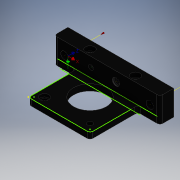
# Autodesk Inventor part: Part1
Saved by Autodesk Inventor 2016 SP1 (Build 200210100, 210)
## iProperties
Created: 2015-12-23
Part Number: Part1
Material: Generic
Document SubType Name: Modeling
Designer: Dirk Alferink
Density: 1 g/cm^3
Appearance: Smooth - Black
Author: Dirk Alferink
Autodesk Inventor part; units mm, degrees
ref_plane "YZ Plane" through (0, 0, 0) normal (1, 0, 0) x (0, 1, 0)
ref_plane "XZ Plane" through (0, 0, 0) normal (0, 1, 0) x (-1, 0, 0)
sketch "Sketch1" plane through (0, 0, 0) normal (0, 0, 1) x (1, 0, 0)
  line L0 (0, 0) -> (42, 0)
  line L1 (42, 0) -> (42, 42)
  line L2 (42, 42) -> (0, 42)
  line L3 (0, 42) -> (0, 0)
  dimension "d0" = 42
  dimension "d1" = 42
  constraints: 8 end point, 2 parallel, 1 horizontal, 1 perpendicular
  measures "d0" distance of L2.end L1.end
  measures "d1" distance of L1.end L0.end
extrude "Extrusion1" add sketch "Sketch1" along normal blind 4.3
sketch "Sketch2" plane through (0, 0, 4.3) normal (0, 0, 1) x (1, 0, 0)
  line L0 (0, 42) -> (0, 0) projected
  line L1 (42, 0) -> (42, 42) projected
  line L2 (0, 42) -> (42, 42)
  line L3 (42, 42) -> (42, 32.6)
  line L4 (42, 32.6) -> (0, 32.6)
  line L5 (0, 32.6) -> (0, 42)
  dimension "d4" = 9.4
  constraints: 8 end point, 2 parallel, 1 horizontal, 1 perpendicular, 1 point on line
  measures "d4" distance of L2.end L3.end
extrude "Extrusion2" add sketch "Sketch2" along normal blind 12.7
sketch "Sketch3" plane through (0, 0, 4.3) normal (0, 0, 1) x (1, 0, 0)
  line L0 (0, 32.6) -> (0, 0) projected
  line L1 (0, 0) -> (42, 0) projected
  point P0 (21, 21)
  dimension "d7" = 21
  dimension "d8" = 21
  measures "d7" distance from line of L0 point (21, 21)
  measures "d8" distance from line of L1 point (21, 21)
hole "Hole1" at (21, 21, 4.3) direction (0, 0, -1) diameter 22.3 end through all
sketch "Sketch4" plane through (0, 0, 17) normal (0, 0, 1) x (1, 0, 0)
  line L0 (42, 42) -> (0, 42) projected
  line L1 (0, 42) -> (0, 32.6) projected
  line L2 (42, 32.6) -> (42, 42) projected
  line L3 (0, 0) -> (42, 0) projected
  point P0 (5.5, 36.5)
  point P1 (36.5, 36.5)
  dimension "d16" = 5.5
  dimension "d17" = 5.5
  dimension "d18" = 5.5
  dimension "d21" = 5.5
  measures "d16" distance from line of L0 point (5.5, 36.5)
  measures "d17" distance from line of L1 point (5.5, 36.5)
  measures "d18" distance from line of L2 point (36.5, 36.5)
  measures "d21" distance from line of point (36.5, 36.5) L0
hole "Hole2" at (5.5, 36.5, 17) at (36.5, 36.5, 17) direction (0, 0, -1) diameter 3.5 end through all counterbore diameter 6 counterbore depth 3
sketch "Sketch5" plane through (0, 0, 4.3) normal (0, 0, 1) x (1, 0, 0)
  line L0 (0, 0) -> (42, 0) projected
  line L1 (0, 32.6) -> (0, 0) projected
  point P0 (5.5, 5.5)
  dimension "d31" = 5.5
  dimension "d32" = 5.5
  measures "d31" distance from line of L0 point (5.5, 5.5)
  measures "d32" distance from line of L1 point (5.5, 5.5)
hole "Hole3" at (5.5, 5.5, 4.3) direction (0, 0, -1) diameter 3.5 end through all counterbore diameter 6 counterbore depth 2
sketch "Sketch6" plane through (0, 0, 4.3) normal (0, 0, 1) x (1, 0, 0)
  line L0 (42, 0) -> (42, 32.6) projected
  line L1 (0, 0) -> (42, 0) projected
  point P0 (36.5, 5.5)
  dimension "d40" = 5.5
  dimension "d41" = 5.5
  measures "d40" distance from line of L0 point (36.5, 5.5)
  measures "d41" distance from line of L1 point (36.5, 5.5)
hole "Hole4" at (36.5, 5.5, 4.3) direction (0, 0, -1) diameter 3.5 end through all
sketch "Sketch7" plane through (0, 42, 0) normal (0, 1, 0) x (1, 0, 0)
  line L0 (0, -17) -> (42, -17) projected
  line L1 (42, 0) -> (42, -17) projected
  point P0 (0, 0)
  point P1 (27, -10.5)
  dimension "d49" = 6.5
  dimension "d50" = 15
  measures "d49" distance from line of L0 point (27, -10.5)
  measures "d50" distance from line of L1 point (27, -10.5)
hole "Hole5" at (27, 42, 10.5) direction (0, -1, 0) diameter 4.917 end through all thread size "M6x1" class "6H" standard "ISO Metric profile"
sketch "Sketch8" plane through (0, 42, 0) normal (0, 1, 0) x (1, 0, 0)
  line L0 (42, -17) -> (0, -17) projected
  line L1 (0, -4.3) -> (0, -17) projected
  point P0 (0, 0)
  point P1 (10, -10.5)
  dimension "d58" = 6.5
  dimension "d59" = 10
  measures "d58" distance from line of L0 point (10, -10.5)
  measures "d59" distance from line of L1 point (10, -10.5)
hole "Hole6" at (10, 42, 10.5) direction (0, -1, 0) diameter 3.242 end through all counterbore diameter 7.5 counterbore depth 2.5 thread size "M4x0.7" class "6H" standard "ISO Metric profile"
sketch "Sketch9" plane through (42, 0, 0) normal (1, 0, 0) x (0, 0, -1)
  line L0 (-17, 32.6) -> (-17, 42) projected
  line L1 (0, 32.6) -> (-17, 32.6)
  line L2 (0, 42) -> (-17, 42) projected
  line L3 (0, 0) -> (0, 42)
  constraints: 4 end point, 1 point on line
extrude "Extrusion3" add sketch "Sketch9" along normal blind 15
sketch "Sketch10" plane through (0, 32.6, 4.3) normal (0, -1, 0) x (1, 0, 0)
  circle A0 centre (50, 4.2) radius 2.5
  line L0 (0, 12.7) -> (57, 12.7) projected
  line L1 (57, 12.7) -> (57, -4.3) projected
  point P0 (0, -4.3)
  dimension "d70" = 5
  dimension "d71" = 8.5
  dimension "d72" = 17
  dimension "d73" = 7
  constraints: 1 centre point
  measures "d70" diameter of A0
  measures "d71" distance from line of L0 A0.centre
  measures "d72" distance of L0.end L1.end
  measures "d73" distance from line of L1 A0.centre
hole "Hole7" at (50, 32.6, 8.5) direction (0, 1, 0) diameter 5 end through all
ref_plane "Work Plane1" through (21, 0, 4.3) normal (1, 0, 0) x (0, 0, -1)
mirror "Mirror1" about plane through (21, 0, 4.3) normal (1, 0, 0) of "Hole7", "Extrusion3"
fillet "Fillet2" radius 2 6 edges at (-15, 32.6, 8.5) (0, 32.6, 2.15) (0, 0, 2.15) (42, 0, 2.15) (42, 32.6, 2.15) (57, 32.6, 8.5)
sketch "Sketch11" plane through (0, 0, 4.3) normal (0, 0, 1) x (1, 0, 0)
  line L0 (-6.1242, 27.6) -> (48.7334, 27.6)
  line L1 (55, 32.6) -> (-13, 32.6)
  line L2 (0, 27.6) -> (0, 2)
  arc A0 (0, 2) -> (2, 0) centre (2, 2) ccw
  line L3 (2, 0) -> (40, 0)
  arc A1 (40, 0) -> (42, 2) centre (40, 2) ccw
  line L4 (42, 2) -> (42, 27.6)
  point P0 (0, 0)
  dimension "d82" = 5
  constraints: 10 end point, 4 point on circle, 2 centre point, 2 point on line, 1 horizontal
  measures "d82" distance between parallel lines of L1 L0
equation "\"d71\" = 0.5 * d72"
body "Solid1"
